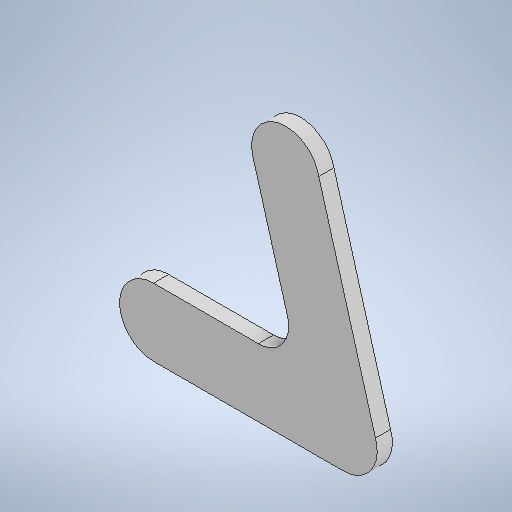
# Autodesk Inventor part: rocker
Saved by Autodesk Inventor 2025.2 (Build 292293000, 293)
## iProperties
Created: 2025-02-15
Part Number: rocker
Material: Generic
Document SubType Name: Modeling
Designer: kenne
Density: 1 g/cm^3
Appearance: Default
Author: kenne
Autodesk Inventor part; units mm, degrees
ref_plane "YZ Plane" through (0, 0, 0) normal (1, 0, 0) x (0, 1, 0)
ref_plane "XZ Plane" through (0, 0, 0) normal (0, 1, 0) x (-1, 0, 0)
ref_plane "XY Plane" through (0, 0, 0) normal (0, 0, 1) x (1, 0, 0)
sketch "Sketch1" plane through (0, 0, 0) normal (0, 0, 1) x (1, 0, 0)
  line L0 (0, 0) -> (125.3, 0)
  line L1 (125.3, 0) -> (0, 0)
  arc A0 (0, 44.72) -> (0, 0) centre (0, 22.36) ccw
  line L2 (0, 44.72) -> (69.214, 44.72)
  arc A1 (69.214, 44.72) -> (88.7387, 69.0544) centre (69.214, 64.72) ccw
  line L3 (88.7387, 69.0544) -> (65.6944, 149.6318)
  arc A2 (109.0995, 160.2579) -> (65.6944, 149.6318) centre (87.1925, 155.78) ccw
  arc A3 (125.3, 0) -> (146.5284, 29.3832) centre (125.3, 22.36) ccw
  line L4 (146.5284, 29.3832) -> (109.0995, 160.2579)
  dimension "d0" = 125.3
  dimension "d1" = 22.36
  dimension "d2" = 20
  dimension "d3" = 74.04
  dimension "d4" = 22.36
  dimension "d5" = 22.36
  dimension "d7" = 133.42
  constraints: 10 end point, 8 point on circle, 5 tangent, 4 centre point, 2 parallel, 1 collinear, 1 horizontal
  measures "d0" distance of L0.start L0.end
  measures "d1" radius of A0
  measures "d2" radius of A1
  measures "d3" angle of L2 L3
  measures "d4" radius of A2
  measures "d5" radius of A3
  measures "d7" vertical distance of A3.centre A2.centre
extrude "Extrusion1" add sketch "Sketch1" along normal blind 10
body "Solid1"
